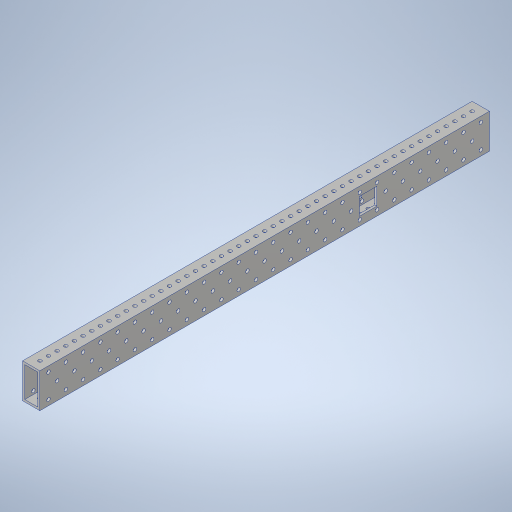
# Autodesk Inventor part: DB1-002
Saved by Autodesk Inventor 2023.4 (Build 274418000, 418)
## iProperties
RuleStatus: InUse
Created: 2025-01-09
Part Number: DB1-002
Material: Aluminum 6061
Document SubType Name: Modeling
Designer: mavericks
Mass: 304.185 g
Surface Area: 718.547 cm^2
Volume: 112.661 cm^3
Density: 2.7 g/cm^3
Appearance: Aluminum - Flat
AfterDocNew0: SHOW
AfterDocOpen0: SHOW
Author: mavericks
Autodesk Inventor part; units mm, degrees
ref_plane "YZ Plane" through (0, 0, 0) normal (1, 0, 0) x (0, 1, 0)
ref_plane "XZ Plane" through (0, 0, 0) normal (0, 1, 0) x (-1, 0, 0)
ref_plane "XY Plane" through (0, 0, 0) normal (0, 0, 1) x (1, 0, 0)
sketch "Sketch1" plane through (0, 0, 0) normal (0, 0, 1) x (1, 0, 0)
  line L0 (-12.7, -25.4) -> (12.7, -25.4)
  line L1 (12.7, -25.4) -> (12.7, 25.4)
  line L2 (12.7, 25.4) -> (-12.7, 25.4)
  line L3 (-12.7, 25.4) -> (-12.7, -25.4)
  line L4 (-12.7, -25.4) -> (12.7, 25.4) construction
  line L5 (12.7, -25.4) -> (-12.7, 25.4) construction
  line L6 (-9.525, 22.225) -> (9.525, 22.225)
  line L7 (9.525, 22.225) -> (9.525, -22.225)
  line L8 (9.525, -22.225) -> (-9.525, -22.225)
  line L9 (-9.525, -22.225) -> (-9.525, 22.225)
  point P0 (0, 0)
  dimension "width" = 25.4
  dimension "height" = 50.8
  dimension "thickness" = 3.175
  constraints: 20 end point, 4 parallel, 2 midpoint, 2 perpendicular, 1 horizontal, 3 other
  measures "width" distance of L2.end L1.end
  measures "height" distance of L1.end L0.end
  measures "thickness" distance between parallel lines of L2 L6
extrude "Extrusion1" add sketch "Sketch1" along normal mid plane 660.4
sketch "Sketch2" plane through (-12.7, 25.4, 330.2) normal (0, 1, 0) x (1, 0, 0)
  line L0 (12.7, 342.9) -> (12.7, 317.5) construction
  line L1 (0, 660.4) -> (0, 0) construction
  point P0 (12.7, 330.2)
  point P1 (12.7, 330.2)
  point P2 (12.7, 304.8)
  point P3 (12.7, 292.1)
  point P4 (12.7, 279.4)
  point P5 (12.7, 266.7)
  point P6 (12.7, 254)
  point P7 (12.7, 241.3)
  point P8 (12.7, 228.6)
  point P9 (12.7, 215.9)
  point P10 (12.7, 203.2)
  point P11 (12.7, 190.5)
  point P12 (12.7, 177.8)
  point P13 (12.7, 165.1)
  point P14 (12.7, 152.4)
  point P15 (12.7, 139.7)
  point P16 (12.7, 127)
  point P17 (12.7, 114.3)
  point P18 (12.7, 101.6)
  point P19 (12.7, 88.9)
  point P20 (12.7, 76.2)
  point P21 (12.7, 63.5)
  point P22 (12.7, 50.8)
  point P23 (12.7, 38.1)
  point P24 (12.7, 25.4)
  point P25 (12.7, 355.6)
  point P26 (12.7, 368.3)
  point P27 (12.7, 381)
  point P28 (12.7, 393.7)
  point P29 (12.7, 406.4)
  point P30 (12.7, 419.1)
  point P31 (12.7, 431.8)
  point P32 (12.7, 444.5)
  point P33 (12.7, 457.2)
  point P34 (12.7, 469.9)
  point P35 (12.7, 482.6)
  point P36 (12.7, 495.3)
  point P37 (12.7, 508)
  point P38 (12.7, 520.7)
  point P39 (12.7, 533.4)
  point P40 (12.7, 546.1)
  point P41 (12.7, 558.8)
  point P42 (12.7, 571.5)
  point P43 (12.7, 584.2)
  point P44 (12.7, 596.9)
  point P45 (12.7, 609.6)
  point P46 (12.7, 622.3)
  point P47 (12.7, 635)
  point P48 (12.7, 330.2)
  point P49 (12.7, 647.7)
  point P50 (12.7, 12.7)
  dimension "d6" = 25.4
  dimension "d9" = 12.7
  dimension "d16" = 12.7
  constraints: 3 vertical, 2 coincident, 2 end point, 2 vertical alignment, 1 midpoint, 48 other
  measures "d6" distance of L0.start L0.end
  measures "d9" distance of L0.end point (12.7, 304.8)
  measures "d16" distance of L0.start point (12.7, 355.6)
hole "Hole1" at (0, 25.4, 12.7) at (0, 25.4, -12.7) at (0, 25.4, 25.4) at (0, 25.4, 38.1) at (0, 25.4, 50.8) at (0, 25.4, 63.5) at (0, 25.4, 76.2) at (0, 25.4, 88.9) at (0, 25.4, 101.6) at (0, 25.4, 114.3) at (0, 25.4, 127) at (0, 25.4, 139.7) at (0, 25.4, 152.4) at (0, 25.4, 165.1) at (0, 25.4, 177.8) at (0, 25.4, 190.5) at (0, 25.4, 203.2) at (0, 25.4, 215.9) at (0, 25.4, 228.6) at (0, 25.4, 241.3) at (0, 25.4, 254) at (0, 25.4, 266.7) at (0, 25.4, 279.4) at (0, 25.4, 292.1) at (0, 25.4, 304.8) at (0, 25.4, -25.4) at (0, 25.4, -38.1) at (0, 25.4, -50.8) at (0, 25.4, -63.5) at (0, 25.4, -76.2) at (0, 25.4, -88.9) at (0, 25.4, -101.6) at (0, 25.4, -114.3) at (0, 25.4, -127) at (0, 25.4, -139.7) at (0, 25.4, -152.4) at (0, 25.4, -165.1) at (0, 25.4, -177.8) at (0, 25.4, -190.5) at (0, 25.4, -203.2) at (0, 25.4, -215.9) at (0, 25.4, -228.6) at (0, 25.4, -241.3) at (0, 25.4, -254) at (0, 25.4, -266.7) at (0, 25.4, -279.4) at (0, 25.4, -292.1) at (0, 25.4, -304.8) at (0, 25.4, 0) at (0, 25.4, 317.5) direction (0, -1, 0) diameter 5.1054 end through all and at (0, 25.4, -317.5) clearance for "Flat Head Machine Screw (82)" size "#10" standard "Ansi Unified Screw Threads"
sketch "Sketch3" plane through (12.7, -25.4, 330.2) normal (1, 0, 0) x (0, 0, -1)
  line L0 (317.5, 42.8625) -> (317.5, 7.9375) construction
  circle A0 centre (317.5, 42.8625) radius 4.7625 construction
  line L1 (0, 47.625) -> (660.4, 47.625) construction
  circle A1 centre (317.5, 7.9375) radius 4.7625 construction
  line L2 (0, 3.175) -> (660.4, 3.175) construction
  line L3 (317.5, 42.8625) -> (342.9, 42.8625) construction
  point P0 (330.2, 25.4)
  point P1 (330.2, 25.4)
  point P2 (342.9, 7.9375)
  point P3 (292.1, 42.8625)
  point P4 (304.8, 25.4)
  point P5 (292.1, 7.9375)
  point P6 (266.7, 42.8625)
  point P7 (279.4, 25.4)
  point P8 (266.7, 7.9375)
  point P9 (241.3, 42.8625)
  point P10 (254, 25.4)
  point P11 (241.3, 7.9375)
  point P12 (215.9, 42.8625)
  point P13 (228.6, 25.4)
  point P14 (215.9, 7.9375)
  point P15 (190.5, 42.8625)
  point P16 (203.2, 25.4)
  point P17 (190.5, 7.9375)
  point P18 (165.1, 42.8625)
  point P19 (177.8, 25.4)
  point P20 (165.1, 7.9375)
  point P21 (139.7, 42.8625)
  point P22 (152.4, 25.4)
  point P23 (139.7, 7.9375)
  point P24 (114.3, 42.8625)
  point P25 (127, 25.4)
  point P26 (114.3, 7.9375)
  point P27 (88.9, 42.8625)
  point P28 (101.6, 25.4)
  point P29 (88.9, 7.9375)
  point P30 (63.5, 42.8625)
  point P31 (76.2, 25.4)
  point P32 (63.5, 7.9375)
  point P33 (38.1, 42.8625)
  point P34 (50.8, 25.4)
  point P35 (38.1, 7.9375)
  point P36 (12.7, 42.8625)
  point P37 (25.4, 25.4)
  point P38 (12.7, 7.9375)
  point P39 (355.6, 25.4)
  point P40 (355.6, 25.4)
  point P41 (368.3, 42.8625)
  point P42 (368.3, 7.9375)
  point P43 (381, 25.4)
  point P44 (381, 25.4)
  point P45 (393.7, 42.8625)
  point P46 (393.7, 7.9375)
  point P47 (406.4, 25.4)
  point P48 (406.4, 25.4)
  point P49 (419.1, 42.8625)
  point P50 (419.1, 7.9375)
  point P51 (431.8, 25.4)
  point P52 (431.8, 25.4)
  point P53 (444.5, 42.8625)
  point P54 (444.5, 7.9375)
  point P55 (457.2, 25.4)
  point P56 (457.2, 25.4)
  point P57 (469.9, 42.8625)
  point P58 (469.9, 7.9375)
  point P59 (482.6, 25.4)
  point P60 (482.6, 25.4)
  point P61 (495.3, 42.8625)
  point P62 (495.3, 7.9375)
  point P63 (508, 25.4)
  point P64 (508, 25.4)
  point P65 (520.7, 42.8625)
  point P66 (520.7, 7.9375)
  point P67 (533.4, 25.4)
  point P68 (533.4, 25.4)
  point P69 (546.1, 42.8625)
  point P70 (546.1, 7.9375)
  point P71 (558.8, 25.4)
  point P72 (558.8, 25.4)
  point P73 (571.5, 42.8625)
  point P74 (571.5, 7.9375)
  point P75 (584.2, 25.4)
  point P76 (584.2, 25.4)
  point P77 (596.9, 42.8625)
  point P78 (596.9, 7.9375)
  point P79 (609.6, 25.4)
  point P80 (609.6, 25.4)
  point P81 (622.3, 42.8625)
  point P82 (622.3, 7.9375)
  point P83 (635, 25.4)
  point P84 (635, 25.4)
  point P85 (647.7, 42.8625)
  point P86 (647.7, 7.9375)
  dimension "d28" = 12.7
  dimension "d29" = 9.525
  dimension "d30" = 9.525
  dimension "d31" = 25.4
  dimension "d34" = 25.4
  dimension "d41" = 25.4
  constraints: 17 coincident, 4 end point, 3 horizontal, 2 centre point, 2 horizontal alignment, 2 tangent, 2 vertical alignment, 1 vertical, 84 other
  measures "d28" horizontal distance of point (330.2, 25.4) L0.start
  measures "d29" diameter of A0
  measures "d30" diameter of A1
  measures "d31" distance of L3.end L3.start
  measures "d34" distance of L0.start point (292.1, 42.863)
  measures "d41" distance of point (330.2, 25.4) point (355.6, 25.4)
hole "Hole2" at (12.7, 0, 0) at (12.7, 17.4625, 12.7) at (12.7, 17.4625, -12.7) at (12.7, -17.4625, -12.7) at (12.7, -17.4625, 12.7) at (12.7, 17.4625, 38.1) at (12.7, 0, 25.4) at (12.7, -17.4625, 38.1) at (12.7, 17.4625, 63.5) at (12.7, 0, 50.8) at (12.7, -17.4625, 63.5) at (12.7, 17.4625, 88.9) at (12.7, 0, 76.2) at (12.7, -17.4625, 88.9) at (12.7, 17.4625, 114.3) at (12.7, 0, 101.6) at (12.7, -17.4625, 114.3) at (12.7, 17.4625, 139.7) at (12.7, 0, 127) at (12.7, -17.4625, 139.7) at (12.7, 17.4625, 165.1) at (12.7, 0, 152.4) at (12.7, -17.4625, 165.1) at (12.7, 17.4625, 190.5) at (12.7, 0, 177.8) at (12.7, -17.4625, 190.5) at (12.7, 17.4625, 215.9) at (12.7, 0, 203.2) at (12.7, -17.4625, 215.9) at (12.7, 17.4625, 241.3) at (12.7, 0, 228.6) at (12.7, -17.4625, 241.3) at (12.7, 17.4625, 266.7) at (12.7, 0, 254) at (12.7, -17.4625, 266.7) at (12.7, 17.4625, 292.1) at (12.7, 0, 279.4) at (12.7, -17.4625, 292.1) at (12.7, 17.4625, 317.5) at (12.7, 0, 304.8) at (12.7, -17.4625, 317.5) at (12.7, 0, -25.4) at (12.7, 17.4625, -38.1) at (12.7, -17.4625, -38.1) at (12.7, 0, -50.8) at (12.7, 17.4625, -63.5) at (12.7, -17.4625, -63.5) at (12.7, 0, -76.2) at (12.7, 17.4625, -88.9) at (12.7, -17.4625, -88.9) direction (-1, 0, 0) diameter 5.1054 end through all and at (12.7, 0, -101.6) (12.7, 17.4625, -114.3) (12.7, -17.4625, -114.3) (12.7, 0, -127) (12.7, 17.4625, -139.7) (12.7, -17.4625, -139.7) (12.7, 0, -152.4) (12.7, 17.4625, -165.1) (12.7, -17.4625, -165.1) (12.7, 0, -177.8) (12.7, 17.4625, -190.5) (12.7, -17.4625, -190.5) (12.7, 0, -203.2) (12.7, 17.4625, -215.9) (12.7, -17.4625, -215.9) (12.7, 0, -228.6) (12.7, 17.4625, -241.3) (12.7, -17.4625, -241.3) (12.7, 0, -254) (12.7, 17.4625, -266.7) (12.7, -17.4625, -266.7) (12.7, 0, -279.4) (12.7, 17.4625, -292.1) (12.7, -17.4625, -292.1) (12.7, 0, -304.8) (12.7, 17.4625, -317.5) (12.7, -17.4625, -317.5) clearance for "Flat Head Machine Screw (82)" size "#10" standard "Ansi Unified Screw Threads"
sketch "Sketch4" plane through (12.7, -25.4, 330.2) normal (1, 0, 0) x (0, 0, -1)
  line L0 (469.759, 38.1) -> (495.159, 38.1)
  line L1 (495.159, 38.1) -> (495.159, 12.7)
  line L2 (495.159, 12.7) -> (469.759, 12.7)
  line L3 (469.759, 12.7) -> (469.759, 38.1)
  line L4 (469.759, 38.1) -> (495.159, 12.7) construction
  line L5 (495.159, 38.1) -> (469.759, 12.7) construction
  line L6 (660.4, 50.8) -> (0, 50.8) projected
  line L7 (660.4, 50.8) -> (660.4, 0) projected
  point P0 (330.2, 25.4)
  point P1 (482.459, 25.4)
  dimension "d53" = 25.4
  dimension "d54" = 25.4
  dimension "d55" = 12.7
  dimension "d56" = 165.2411
  constraints: 12 end point, 2 midpoint, 2 parallel, 1 horizontal, 1 perpendicular
  measures "d53" distance of L1.end L2.end
  measures "d54" distance of L0.end L1.end
  measures "d55" distance between parallel lines of L6 L0
  measures "d56" distance between parallel lines of L7 L1
extrude "Extrusion2" cut sketch "Sketch4" against normal blind 25.4
body "Solid1"
